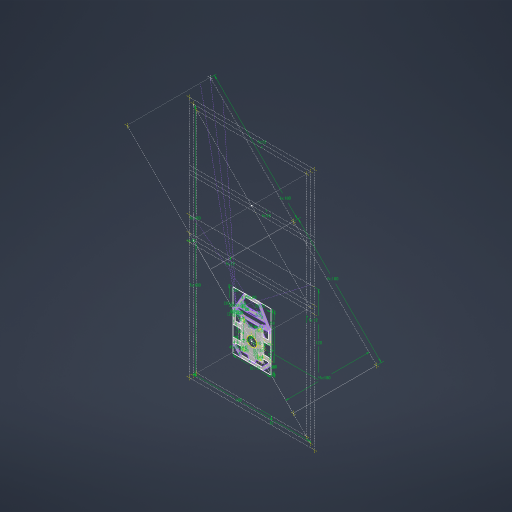
# Autodesk Inventor part: chassis
Saved by Autodesk Inventor 2023.5 (Build 275446000, 446)
## iProperties
Created: 2025-01-19
Part Number: chassis
Material: 一般
Document SubType Name: Modeling
Designer: IshiiLabHonda
Density: 1 g/cm^3
Appearance: 既定
Author: IshiiLabHonda
Autodesk Inventor part; units mm, degrees
ref_plane "YZ Plane" through (0, 0, 0) normal (1, 0, 0) x (0, 1, 0)
ref_plane "XZ Plane" through (0, 0, 0) normal (0, 1, 0) x (-1, 0, 0)
ref_plane "XY Plane" through (0, 0, 0) normal (0, 0, 1) x (1, 0, 0)
sketch "スケッチ1" plane through (0, 0, 0) normal (0, 0, 1) x (1, 0, 0)
  line L0 (-90, 90) -> (90, 90) construction
  line L1 (90, 90) -> (90, -90) construction
  line L2 (90, -90) -> (-90, -90) construction
  line L3 (-90, -90) -> (-90, 90) construction
  line L4 (-90, 90) -> (-90, 270) construction
  line L5 (-90, 270) -> (90, 270) construction
  line L6 (90, 270) -> (90, 90) construction
  line L7 (-90, 90) -> (90, -90) construction
  line L8 (90, 90) -> (-90, -90) construction
  line L9 (0, 0) -> (0, 10) construction
  line L10 (0, 0) -> (10, 0) construction
  line L11 (-90, 270) -> (90, 90) construction
  line L12 (-90, 90) -> (90, 270) construction
  line L13 (-96, 276) -> (96, 276) construction
  line L14 (96, 276) -> (96, -96) construction
  line L15 (96, -96) -> (-96, -96) construction
  line L16 (-96, -96) -> (-96, 276) construction
  line L17 (-84, 264) -> (84, 264) construction
  line L18 (84, 264) -> (84, -84) construction
  line L19 (84, -84) -> (-84, -84) construction
  line L20 (-84, -84) -> (-84, 264) construction
  line L21 (-96, 96) -> (96, 96) construction
  line L22 (-96, 84) -> (96, 84) construction
  line L23 (-63.6396, 63.6396) -> (63.6396, 190.9188) construction
  line L24 (63.6396, 190.9188) -> (190.9188, 63.6396) construction
  line L25 (190.9188, 63.6396) -> (63.6396, -63.6396) construction
  line L26 (63.6396, -63.6396) -> (-63.6396, 63.6396) construction
  line L27 (-190.9188, 190.9188) -> (-63.6396, 318.1981) construction
  line L28 (-63.6396, 318.1981) -> (63.6396, 190.9188) construction
  line L29 (-63.6396, 63.6396) -> (-190.9188, 190.9188) construction
  line L30 (-96, 120) -> (96, 120) construction
  line L31 (-96, 186) -> (96, 186) construction
  line L32 (-96, 174) -> (96, 174) construction
  line L33 (-96, 180) -> (96, 180) construction
  point P0 (-63.6396, 318.1981)
  point P1 (-90, 120)
  point P2 (90, 120)
  point P3 (0, 180)
  dimension "d8" = 10
  dimension "d9" = 10
  dimension "d10" = 12
  dimension "d11" = 12
  dimension "d12" = 12
  dimension "d13" = 12
  dimension "d14" = 180
  dimension "d15" = 180
  dimension "d16" = 180
  dimension "d17" = 12
  dimension "d34" = 180
  dimension "d35" = 180
  dimension "d36" = 180
  dimension "d37" = 120
  dimension "d85" = 12
  constraints: 68 end point, 16 parallel, 16 point on line, 9 perpendicular, 4 midpoint, 3 coincident, 1 horizontal, 7 other
  measures "d8" distance of L9.start L9.end
  measures "d9" distance of L9.start L10.end
  measures "d10" distance between parallel lines of L15 L19
  measures "d11" distance between parallel lines of L16 L20
  measures "d12" distance between parallel lines of L14 L18
  measures "d13" distance between parallel lines of L17 L13
  measures "d14" distance of L1.end L2.end
  measures "d15" distance of L2.end L0.start
  measures "d16" distance between parallel lines of L0 L5
  measures "d17" distance between parallel lines of L22 L21
  measures "d34" distance between parallel lines of L26 L24
  measures "d35" distance of L23.end L24.end
  measures "d36" distance between parallel lines of L23 L27
  measures "d37" distance between parallel lines of L10 L30
  measures "d85" distance between parallel lines of L32 L31
sketch "スケッチ2" plane through (0, 0, 0) normal (0, 0, 1) x (1, 0, 0)
  line L0 (63.6396, 190.9188) -> (190.9188, 63.6396) construction
  line L1 (-63.6396, 318.1981) -> (63.6396, 190.9188) construction
  line L2 (-84, 264) -> (84, 264) construction
  line L3 (-90, 270) -> (90, 270) construction
  line L4 (90, 270) -> (90, 90) construction
  line L5 (-96, 276) -> (96, 276) construction
  line L6 (-90, 90) -> (90, 270) construction
  line L7 (-90, 270) -> (90, 90) construction
  line L8 (-63.6396, 63.6396) -> (63.6396, 190.9188) construction
  line L9 (-96, 120) -> (96, 120) construction
  line L10 (-90, 90) -> (90, 90) construction
  line L11 (-96, 96) -> (96, 96) construction
  line L12 (-96, 84) -> (96, 84) construction
  line L13 (90, -90) -> (-90, -90) construction
  line L14 (0, 0) -> (0, 10) construction
  line L15 (0, 0) -> (10, 0) construction
  line L16 (190.9188, 63.6396) -> (63.6396, -63.6396) construction
  line L17 (63.6396, -63.6396) -> (-63.6396, 63.6396) construction
  line L18 (84, -84) -> (-84, -84) construction
  line L19 (96, -96) -> (-96, -96) construction
  line L20 (-90, 90) -> (-90, 270) construction
  line L21 (-63.6396, 63.6396) -> (-190.9188, 190.9188) construction
  line L22 (-190.9188, 190.9188) -> (-63.6396, 318.1981) construction
  line L23 (96, 276) -> (96, -96) construction
  line L24 (-96, -96) -> (-96, 276) construction
  line L25 (84, 264) -> (84, -84) construction
  line L26 (-84, -84) -> (-84, 264) construction
  line L27 (90, 90) -> (90, -90) construction
  line L28 (-90, 90) -> (90, -90) construction
  line L29 (90, 90) -> (-90, -90) construction
  line L30 (-90, -90) -> (-90, 90) construction
  circle A0 centre (0, 0) radius 16 construction
  circle A1 centre (0, 0) radius 7.5 construction
  line L31 (20, 11.5) -> (28.75, 11.5) construction
  line L32 (28.75, 11.5) -> (28.75, -11.5) construction
  line L33 (28.75, -11.5) -> (20, -11.5) construction
  line L34 (20, -11.5) -> (20, 11.5) construction
  line L35 (20, 11.5) -> (18, 11.5) construction
  line L36 (18, 11.5) -> (18, -11.5) construction
  line L37 (18, -11.5) -> (20, -11.5) construction
  line L38 (18, 1.5) -> (17, 1.5) construction
  line L39 (17, -1.5) -> (18, -1.5) construction
  line L40 (-17, 26) -> (17, 26) construction
  line L41 (17, 26) -> (17, -20) construction
  line L42 (17, -20) -> (-17, -20) construction
  line L43 (-17, -20) -> (-17, 26) construction
  line L44 (-20, 11.5) -> (-28.75, 11.5) construction
  line L45 (-28.75, 11.5) -> (-28.75, -11.5) construction
  line L46 (-28.75, -11.5) -> (-20, -11.5) construction
  line L47 (-20, -11.5) -> (-20, 11.5) construction
  line L48 (-20, 11.5) -> (-18, 11.5) construction
  line L49 (-18, 11.5) -> (-18, -11.5) construction
  line L50 (-18, -11.5) -> (-20, -11.5) construction
  line L51 (-18, 1.5) -> (-17, 1.5) construction
  line L52 (-17, -1.5) -> (-18, -1.5) construction
  line L53 (-14.5, 26) -> (-14.5, -20) construction
  line L54 (14.5, 26) -> (14.5, -20) construction
  line L55 (-10.5, 26) -> (-10.5, 21) construction
  line L56 (-10.5, 21) -> (-14.5, 21) construction
  line L57 (-14.5, 26) -> (-10.5, 21) construction
  line L58 (-10.5, 26) -> (-14.5, 21) construction
  circle A2 centre (-12.5, 23.5) radius 1 construction
  line L59 (10.5, 26) -> (10.5, 21) construction
  line L60 (10.5, 21) -> (14.5, 21) construction
  line L61 (10.5, 26) -> (14.5, 21) construction
  line L62 (10.5, 21) -> (14.5, 26) construction
  circle A3 centre (12.5, 23.5) radius 1 construction
  line L63 (-14.5, -15) -> (-10.5, -15) construction
  line L64 (-10.5, -15) -> (-10.5, -20) construction
  line L65 (10.5, -20) -> (10.5, -15) construction
  line L66 (10.5, -15) -> (14.5, -15) construction
  line L67 (-14.5, -15) -> (-10.5, -20) construction
  line L68 (-10.5, -15) -> (-14.5, -20) construction
  circle A4 centre (-12.5, -17.5) radius 1 construction
  line L69 (10.5, -15) -> (14.5, -20) construction
  line L70 (14.5, -15) -> (10.5, -20) construction
  circle A5 centre (12.5, -17.5) radius 1 construction
  point P0 (90, 120)
  point P1 (-90, 120)
  point P2 (-63.6396, 318.1981)
  point P3 (-12.5, -17.5)
  dimension "d38" = 32
  dimension "d39" = 15
  dimension "d40" = 8.75
  dimension "d41" = 2
  dimension "d42" = 23
  dimension "d44" = 3
  dimension "d45" = 1
  dimension "d48" = 2.5
  dimension "d49" = 20
  dimension "d50" = 26
  dimension "d51" = 2
  dimension "d52" = 5
  dimension "d53" = 4
  dimension "d54" = 2
  dimension "d55" = 4
  dimension "d56" = 5
  dimension "d57" = 2
  dimension "d58" = 4
  dimension "d59" = 5
  dimension "d60" = 2
  dimension "d61" = 5
  dimension "d62" = 4
  dimension "d63" = 57.5
  dimension "d71" = 41
  dimension "d154" = 29
  constraints: 80 end point, 18 point on line, 12 parallel, 10 symmetric about line, 6 centre point, 6 midpoint, 6 perpendicular, 2 coincident, 2 collinear, 5 other
  measures "d38" diameter of A0
  measures "d39" diameter of A1
  measures "d40" distance between parallel lines of L34 L32
  measures "d41" distance between parallel lines of L36 L34
  measures "d42" distance between parallel lines of L33 L31
  measures "d44" distance between parallel lines of L39 L38
  measures "d45" distance between parallel lines of L41 L36
  measures "d48" distance between parallel lines of L43 L53
  measures "d49" distance between parallel lines of L42 L15
  measures "d50" distance between parallel lines of L15 L40
  measures "d51" diameter of A2
  measures "d52" distance of L55.start L55.end
  measures "d53" distance of L55.end L56.end
  measures "d54" diameter of A3
  measures "d55" distance of L59.end L60.end
  measures "d56" distance of L59.start L59.end
  measures "d57" diameter of A4
  measures "d58" distance of L63.start L63.end
  measures "d59" distance of L63.end L64.end
  measures "d60" diameter of A5
  measures "d61" distance of L65.start L65.end
  measures "d62" distance of L65.end L66.end
  measures "d63" distance between parallel lines of L32 L45
  measures "d71" distance of point (-12.5, -17.5) point (-12.5, 23.5)
  measures "d154" distance between parallel lines of L54 L53
sketch "スケッチ3" plane through (0, 0, 0) normal (0, 0, 1) x (1, 0, 0)
  line L0 (63.6396, 190.9188) -> (190.9188, 63.6396) construction
  line L1 (-63.6396, 318.1981) -> (63.6396, 190.9188) construction
  line L2 (-84, 264) -> (84, 264) construction
  line L3 (-90, 270) -> (90, 270) construction
  line L4 (90, 270) -> (90, 90) construction
  line L5 (-96, 276) -> (96, 276) construction
  line L6 (-90, 90) -> (90, 270) construction
  line L7 (-90, 270) -> (90, 90) construction
  line L8 (-63.6396, 63.6396) -> (63.6396, 190.9188) construction
  line L9 (-96, 120) -> (96, 120) construction
  line L10 (-90, 90) -> (90, 90) construction
  line L11 (-96, 96) -> (96, 96) construction
  line L12 (-96, 84) -> (96, 84) construction
  line L13 (90, -90) -> (-90, -90) construction
  line L14 (0, 0) -> (0, 10) construction
  line L15 (0, 0) -> (10, 0) construction
  line L16 (190.9188, 63.6396) -> (63.6396, -63.6396) construction
  line L17 (63.6396, -63.6396) -> (-63.6396, 63.6396) construction
  line L18 (84, -84) -> (-84, -84) construction
  line L19 (96, -96) -> (-96, -96) construction
  line L20 (-90, 90) -> (-90, 270) construction
  line L21 (-63.6396, 63.6396) -> (-190.9188, 190.9188) construction
  line L22 (-190.9188, 190.9188) -> (-63.6396, 318.1981) construction
  line L23 (96, 276) -> (96, -96) construction
  line L24 (-96, -96) -> (-96, 276) construction
  line L25 (84, 264) -> (84, -84) construction
  line L26 (-84, -84) -> (-84, 264) construction
  line L27 (90, 90) -> (90, -90) construction
  line L28 (-90, 90) -> (90, -90) construction
  line L29 (90, 90) -> (-90, -90) construction
  line L30 (-90, -90) -> (-90, 90) construction
  line L31 (-18, 1.5) -> (-17, 1.5) construction
  line L32 (-17, -1.5) -> (-18, -1.5) construction
  line L33 (-20, 11.5) -> (-18, 11.5) construction
  line L34 (-28.75, 11.5) -> (-28.75, -11.5) construction
  line L35 (63.6396, -63.6396) -> (-63.6396, 63.6396) construction
  line L36 (84, -84) -> (-84, -84) construction
  line L37 (-90, -90) -> (-90, 90) construction
  line L38 (96, -96) -> (-96, -96) construction
  line L39 (-90, 90) -> (90, 90) construction
  line L40 (90, -90) -> (-90, -90) construction
  line L41 (90, 90) -> (-90, -90) construction
  line L42 (-90, 90) -> (90, -90) construction
  line L43 (90, 90) -> (90, -90) construction
  line L44 (-28.75, -11.5) -> (-20, -11.5) construction
  line L45 (-20, 11.5) -> (-28.75, 11.5) construction
  line L46 (-18, 11.5) -> (-18, -11.5) construction
  line L47 (-18, -11.5) -> (-20, -11.5) construction
  line L48 (0, 0) -> (0, 10) construction
  line L49 (0, 0) -> (10, 0) construction
  circle A0 centre (0, 0) radius 16 construction
  circle A1 centre (0, 0) radius 7.5 projected
  line L50 (-14.5, 26) -> (-14.5, -20) construction
  line L51 (-17, 26) -> (17, 26) construction
  line L52 (-17, -20) -> (-17, 26) construction
  line L53 (17, -20) -> (-17, -20) construction
  line L54 (-14.5, -15) -> (-10.5, -15) construction
  circle A2 centre (-12.5, -17.5) radius 1 projected
  line L55 (-10.5, -15) -> (-14.5, -20) construction
  line L56 (-14.5, -15) -> (-10.5, -20) construction
  line L57 (-63.6396, 318.1981) -> (63.6396, 190.9188) construction
  line L58 (-84, 264) -> (84, 264) construction
  line L59 (-90, 270) -> (90, 270) construction
  line L60 (90, 270) -> (90, 90) construction
  line L61 (-96, 276) -> (96, 276) construction
  line L62 (-90, 90) -> (90, 270) construction
  line L63 (-90, 270) -> (90, 90) construction
  line L64 (-63.6396, 63.6396) -> (63.6396, 190.9188) construction
  line L65 (-96, 120) -> (96, 120) construction
  line L66 (-96, 96) -> (96, 96) construction
  line L67 (-96, 84) -> (96, 84) construction
  line L68 (84, 264) -> (84, -84) construction
  line L69 (96, 276) -> (96, -96) construction
  line L70 (-96, -96) -> (-96, 276) construction
  line L71 (-84, -84) -> (-84, 264) construction
  line L72 (-63.6396, 63.6396) -> (-190.9188, 190.9188) construction
  line L73 (-90, 90) -> (-90, 270) construction
  line L74 (-190.9188, 190.9188) -> (-63.6396, 318.1981) construction
  line L75 (-20, -11.5) -> (-20, 11.5) construction
  line L76 (10.5, -15) -> (14.5, -15) construction
  line L77 (10.5, -20) -> (10.5, -15) construction
  circle A3 centre (12.5, -17.5) radius 1 projected
  line L78 (10.5, -15) -> (14.5, -20) construction
  line L79 (14.5, -15) -> (10.5, -20) construction
  line L80 (-10.5, -15) -> (-10.5, -20) construction
  line L81 (63.6396, 190.9188) -> (190.9188, 63.6396) construction
  line L82 (190.9188, 63.6396) -> (63.6396, -63.6396) construction
  line L83 (20, 11.5) -> (28.75, 11.5) construction
  line L84 (28.75, 11.5) -> (28.75, -11.5) construction
  line L85 (17, -1.5) -> (18, -1.5) construction
  line L86 (18, -11.5) -> (20, -11.5) construction
  line L87 (28.75, -11.5) -> (20, -11.5) construction
  line L88 (14.5, 26) -> (14.5, -20) construction
  line L89 (17, 26) -> (17, -20) construction
  line L90 (18, 11.5) -> (18, -11.5) construction
  line L91 (20, -11.5) -> (20, 11.5) construction
  line L92 (20, 11.5) -> (18, 11.5) construction
  line L93 (18, 1.5) -> (17, 1.5) construction
  line L94 (-10.5, 26) -> (-10.5, 21) construction
  line L95 (10.5, 21) -> (14.5, 21) construction
  circle A4 centre (12.5, 23.5) radius 1 projected
  line L96 (10.5, 26) -> (14.5, 21) construction
  line L97 (10.5, 21) -> (14.5, 26) construction
  line L98 (10.5, 26) -> (10.5, 21) construction
  line L99 (-10.5, 21) -> (-14.5, 21) construction
  circle A5 centre (-12.5, 23.5) radius 1 projected
  line L100 (-14.5, 26) -> (-10.5, 21) construction
  line L101 (-10.5, 26) -> (-14.5, 21) construction
  line L102 (29.25, 58) -> (29.25, -30)
  line L103 (-29.25, -30) -> (-29.25, 58)
  line L104 (-29.25, 8.5) -> (-17, 8.5)
  line L105 (-17, 8.5) -> (-17, -8.5)
  line L106 (-17, -8.5) -> (-29.25, -8.5)
  line L107 (29.25, 8.5) -> (17, 8.5)
  line L108 (17, 8.5) -> (17, -8.5)
  line L109 (17, -8.5) -> (29.25, -8.5)
  line L110 (10.991, 46.9185) -> (16.1478, 42.9616) construction
  line L111 (11.8865, 37.4081) -> (14.2666, 35.5818) construction
  line L112 (14.2666, 35.5818) -> (18.5279, 41.1353) construction
  line L113 (11.9003, 38.658) -> (10.9773, 45.6686) construction
  line L114 (18.5279, 41.1353) -> (16.1478, 42.9616) construction
  line L115 (11.8865, 37.4081) -> (6.7297, 41.365) construction
  line L116 (11.9003, 38.658) -> (7.9335, 41.7018) construction
  line L117 (7.9335, 41.7018) -> (10.9773, 45.6686) construction
  line L118 (6.7297, 41.365) -> (10.991, 46.9185) construction
  line L119 (10.991, 46.9185) -> (11.8865, 37.4081) construction
  line L120 (14.9441, 42.6248) -> (11.9003, 38.658) construction
  line L121 (7.9335, 41.7018) -> (14.9441, 42.6248) construction
  line L122 (6.7297, 41.365) -> (16.1478, 42.9616) construction
  line L123 (16.1478, 42.9616) -> (11.8865, 37.4081) construction
  line L124 (10.9773, 45.6686) -> (14.9441, 42.6248) construction
  line L125 (-25.2554, 25.0784) -> (-25.9466, 30.0304) construction
  line L126 (-20.1078, 31.6026) -> (-18.8984, 22.9366) construction
  line L127 (-20.9946, 30.7216) -> (-20.3034, 25.7696) construction
  line L128 (-25.2554, 25.0784) -> (-20.9946, 30.7216) construction
  line L129 (-25.9466, 30.0304) -> (-20.3034, 25.7696) construction
  line L130 (-27.0406, 30.635) -> (-20.1078, 31.6026) construction
  line L131 (-18.8984, 22.9366) -> (-25.8312, 21.969) construction
  line L132 (-25.8312, 21.969) -> (-27.0406, 30.635) construction
  line L133 (-63.6396, 318.1981) -> (-23.125, 27.9) construction
  line L134 (11.4388, 42.1633) -> (-90, 120) construction
  line L135 (-23.125, 27.9) -> (-78.8228, 303.0149) construction
  line L136 (-23.125, 27.9) -> (-44.1788, 298.7372) construction
  line L137 (-10.9773, 45.6686) -> (-7.9335, 41.7018) construction
  line L138 (-10.991, 46.9185) -> (-6.7297, 41.365) construction
  line L139 (-16.1478, 42.9616) -> (-10.991, 46.9185) construction
  line L140 (-6.7297, 41.365) -> (-16.1478, 42.9616) construction
  line L141 (-14.9441, 42.6248) -> (-7.9335, 41.7018) construction
  line L142 (-14.9441, 42.6248) -> (-10.9773, 45.6686) construction
  line L143 (-16.1478, 42.9616) -> (-18.5279, 41.1353) construction
  line L144 (-7.9335, 41.7018) -> (-11.9003, 38.658) construction
  line L145 (-10.9773, 45.6686) -> (-11.9003, 38.658) construction
  line L146 (-11.9003, 38.658) -> (-14.9441, 42.6248) construction
  line L147 (-10.991, 46.9185) -> (-11.8865, 37.4081) construction
  line L148 (-6.7297, 41.365) -> (-11.8865, 37.4081) construction
  line L149 (-11.8865, 37.4081) -> (-16.1478, 42.9616) construction
  line L150 (-18.5279, 41.1353) -> (-14.2666, 35.5818) construction
  line L151 (-14.2666, 35.5818) -> (-11.8865, 37.4081) construction
  line L152 (-11.4388, 42.1633) -> (90, 120) construction
  circle A6 centre (-8.395, 38.1965) radius 0.625 construction
  circle A7 centre (-8.395, 38.1965) radius 0.8
  circle A8 centre (-8.395, 38.1965) radius 1.5 construction
  circle A9 centre (-15.2072, 39.2717) radius 0.625 construction
  circle A10 centre (-15.2072, 39.2717) radius 0.8
  circle A11 centre (-15.2072, 39.2717) radius 1.5 construction
  line L153 (-20.3034, 25.7696) -> (-25.2554, 25.0784) construction
  line L154 (-26.1422, 24.1974) -> (-19.2094, 25.165) construction
  line L155 (-25.601, 27.5544) -> (-20.649, 28.2456) construction
  line L156 (-22.3648, 22.4528) -> (-22.7794, 25.424) construction
  circle A12 centre (-18.173, 28.5911) radius 1.5 construction
  circle A13 centre (-18.173, 28.5911) radius 0.8
  circle A14 centre (-18.173, 28.5911) radius 0.625 construction
  circle A15 centre (-27.1405, 25.3286) radius 0.8
  circle A16 centre (-27.1405, 25.3286) radius 0.625 construction
  line L157 (-25.9466, 30.0304) -> (-20.9946, 30.7216) construction
  circle A17 centre (8.395, 38.1965) radius 0.625 construction
  circle A18 centre (8.395, 38.1965) radius 0.8
  circle A19 centre (8.395, 38.1965) radius 1.5 construction
  circle A20 centre (15.2072, 39.2717) radius 1.5 construction
  circle A21 centre (15.2072, 39.2717) radius 0.8
  circle A22 centre (15.2072, 39.2717) radius 0.625 construction
  circle A23 centre (18.173, 28.5911) radius 0.625 construction
  circle A24 centre (18.173, 28.5911) radius 0.8
  circle A25 centre (18.173, 28.5911) radius 1.5 construction
  circle A26 centre (27.1405, 25.3286) radius 0.625 construction
  circle A27 centre (27.1405, 25.3286) radius 0.8
  circle A28 centre (27.1405, 25.3286) radius 1.5 construction
  line L158 (-29.25, -30) -> (29.25, -30)
  line L159 (-29.25, 58) -> (29.25, 58)
  line L160 (-11.4388, 42.1633) -> (-8.395, 38.1965) construction
  line L161 (-29.25, 28.2016) -> (-12.0459, 58)
  line L162 (-29.25, -17.6878) -> (-16.9378, -30)
  line L163 (29.25, 28.2016) -> (12.0459, 58)
  line L164 (29.25, -17.6878) -> (16.9378, -30)
  line L165 (-9.7365, 54) -> (9.7365, 54)
  line L166 (9.7365, 54) -> (25.25, 27.1298)
  line L167 (25.25, 27.1298) -> (25.25, 14.5)
  line L168 (25.25, 14.5) -> (17, 14.5)
  line L169 (3.695, 18.0905) -> (-3.695, 18.0905)
  line L170 (-17, 14.5) -> (-25.25, 14.5)
  line L171 (-25.25, 14.5) -> (-25.25, 27.1298)
  line L172 (-25.25, 27.1298) -> (-9.7365, 54)
  line L173 (20.1078, 31.6026) -> (18.8984, 22.9366) construction
  line L174 (20.9946, 30.7216) -> (20.3034, 25.7696) construction
  line L175 (25.9466, 30.0304) -> (20.3034, 25.7696) construction
  line L176 (25.2554, 25.0784) -> (20.9946, 30.7216) construction
  line L177 (27.0406, 30.635) -> (20.1078, 31.6026) construction
  line L178 (25.2554, 25.0784) -> (25.9466, 30.0304) construction
  line L179 (18.8984, 22.9366) -> (25.8312, 21.969) construction
  line L180 (25.8312, 21.969) -> (27.0406, 30.635) construction
  line L181 (20.3034, 25.7696) -> (25.2554, 25.0784) construction
  line L182 (26.1422, 24.1974) -> (19.2094, 25.165) construction
  line L183 (25.9466, 30.0304) -> (20.9946, 30.7216) construction
  line L184 (-9.7365, 22.9366) -> (-9.7365, 26)
  line L185 (9.7365, 22.9366) -> (9.7365, 26)
  line L186 (9.7365, 26) -> (17, 26)
  line L187 (17, 26) -> (17, 14.5)
  line L188 (-9.7365, 26) -> (-17, 26)
  line L189 (-17, 26) -> (-17, 14.5)
  line L190 (-9.7365, 22.9366) -> (-3.695, 18.0905)
  line L191 (9.7365, 22.9366) -> (3.695, 18.0905)
  line L192 (-17, -14.5) -> (-25.25, -14.5)
  line L193 (-25.25, -14.5) -> (-25.25, -16.0309)
  line L194 (-25.25, -16.0309) -> (-15.2809, -26)
  line L195 (-15.2809, -26) -> (15.2809, -26)
  line L196 (15.2809, -26) -> (25.25, -16.0309)
  line L197 (25.25, -16.0309) -> (25.25, -14.5)
  line L198 (25.25, -14.5) -> (17, -14.5)
  line L199 (17, -14.5) -> (17, -20.8804)
  line L200 (17, -20.8804) -> (6.6466, -20.8804)
  line L201 (6.6466, -20.8804) -> (4.5158, -27.0126)
  line L202 (4.5158, -27.0126) -> (-4.5158, -27.0126)
  line L203 (-4.5158, -27.0126) -> (-6.6466, -20.8804)
  line L204 (-6.6466, -20.8804) -> (-17, -20.8804)
  line L205 (-17, -20.8804) -> (-17, -14.5)
  line L206 (-16.1661, 42.8636) -> (16.1661, 42.8636)
  line L207 (-20.6579, 35.0836) -> (20.6579, 35.0836)
  line L208 (-22.045, 32.6811) -> (-12.2942, 28.5594)
  line L209 (-12.2942, 28.5594) -> (12.2942, 28.5594)
  line L210 (12.2942, 28.5594) -> (22.045, 32.6811)
  line L211 (-25.25, 25.1515) -> (25.25, 25.1515)
  circle A29 centre (-27.1405, 25.3286) radius 1.5 construction
  line L212 (-7.5571, 35.0836) -> (-5.0762, 37.1727)
  line L213 (-5.0762, 37.1727) -> (5.0762, 37.1727)
  line L214 (5.0762, 37.1727) -> (7.5571, 35.0836)
  line L215 (-6.2476, 42.8636) -> (0, 41.1322)
  line L216 (0, 41.1322) -> (6.2476, 42.8636)
  line L217 (-17, 18.9574) -> (-20.6579, 14.5)
  line L218 (17, 18.9574) -> (20.6579, 14.5)
  point P0 (29.25, -8.5)
  point P1 (29.25, 8.5)
  point P2 (29.25, -17.6878)
  point P3 (29.25, 28.2016)
  point P4 (16.5079, 42.2717)
  point P5 (9.7365, 25.1515)
  point P6 (-9.7365, 25.1515)
  point P7 (17, 25.1515)
  point P8 (-17, 25.1515)
  point P9 (-4.3925, 58)
  point P10 (4.5158, 58)
  point P11 (4.8676, -26)
  point P12 (-4.8676, -26)
  dimension "d78" = 17
  dimension "d80" = 0.5
  dimension "d81" = 58.5
  dimension "d82" = 57.5
  dimension "d84" = 0
  dimension "d119" = 5
  dimension "d123" = 5
  dimension "d124" = 5
  dimension "d125" = 6.5
  dimension "d126" = 7
  dimension "d127" = 3
  dimension "d128" = 7
  dimension "d130" = 5
  dimension "d131" = 5
  dimension "d132" = 6.5
  dimension "d133" = 7
  dimension "d134" = 3
  dimension "d135" = 105
  dimension "d141" = 1.25
  dimension "d142" = 1.6
  dimension "d143" = 3
  dimension "d144" = 1.25
  dimension "d145" = 1.6
  dimension "d146" = 3
  dimension "d156" = 3
  dimension "d157" = 6.5
  dimension "d158" = 7
  dimension "d161" = 1.25
  dimension "d162" = 1.6
  dimension "d163" = 3
  dimension "d164" = 1.25
  dimension "d165" = 1.6
  dimension "d173" = 5
  dimension "d187" = 88
  dimension "d192" = 2.2094
  dimension "d193" = 58
  dimension "d194" = 30
  dimension "d195" = 30.1
  dimension "d198" = 45
  dimension "d199" = 30
  dimension "d203" = 4
  dimension "d204" = 4
  dimension "d205" = 0
  dimension "d206" = 4
  dimension "d207" = 4
  dimension "d208" = 4
  dimension "d209" = 4
  dimension "d210" = 6
  dimension "d211" = 6
  dimension "d240" = 3
  constraints: 234 end point, 48 horizontal alignment, 37 parallel, 35 point on line, 27 perpendicular, 24 centre point, 17 coincident, 14 midpoint, 11 equal radius, 6 horizontal, 3 tangent, 1 equal length, 18 other
  measures "d78" distance between parallel lines of L106 L104
  measures "d80" distance between parallel lines of L103 L34
  measures "d81" distance between parallel lines of L102 L103
  measures "d82" distance between parallel lines of L84 L34
  measures "d84" distance between parallel lines of L105 L52
  measures "d119" distance between parallel lines of L125 L127
  measures "d123" distance between parallel lines of L120 L117
  measures "d124" distance of L124.end L113.start
  measures "d125" distance between parallel lines of L123 L118
  measures "d126" distance between parallel lines of L110 L115
  measures "d127" distance between parallel lines of L112 L123
  measures "d128" angle of L135 L136
  measures "d130" distance between parallel lines of L146 L137
  measures "d131" distance of L144.end L141.start
  measures "d132" distance between parallel lines of L149 L138
  measures "d133" distance between parallel lines of L148 L139
  measures "d134" distance between parallel lines of L150 L149
  measures "d135" angle of L134 L152
  measures "d141" diameter of A6
  measures "d142" diameter of A7
  measures "d143" diameter of A8
  measures "d144" diameter of A9
  measures "d145" diameter of A10
  measures "d146" diameter of A11
  measures "d156" distance between parallel lines of L131 L153
  measures "d157" distance between parallel lines of L154 L130
  measures "d158" distance between parallel lines of L126 L132
  measures "d161" diameter of A14
  measures "d162" diameter of A13
  measures "d163" diameter of A12
  measures "d164" diameter of A16
  measures "d165" diameter of A15
  measures "d173" distance of L128.start L129.start
  measures "d187" distance between parallel lines of L158 L159
  measures "d192" distance from line of L103 L130.start
  measures "d193" distance of the line from the sketch origin of L159
  measures "d194" distance of the line from the sketch origin of L158
  measures "d195" distance from line of point (-23.125, 27.9) L159
  measures "d198" angle of L103 L162
  measures "d199" angle of L103 L161
  measures "d203" distance between parallel lines of L165 L159
  measures "d204" distance between parallel lines of L161 L172
  measures "d205" distance between parallel lines of L189 L52
  measures "d206" distance between parallel lines of L103 L171
  measures "d207" distance between parallel lines of L158 L195
  measures "d208" distance between parallel lines of L162 L194
  measures "d209" distance between parallel lines of L103 L193
  measures "d210" distance between parallel lines of L192 L106
  measures "d211" distance between parallel lines of L104 L170
  measures "d240" diameter of A29
extrude "押し出し1" add sketch "スケッチ3" against normal blind 1 contours A1 | A2 | A3 | A4 | A5 | L102 L163 L159 | L102 L107 L108 L109 L164 L158 L162 L103 L106 L105 L104 L161 L159 L163 | L102 L109 L108 L107 | L161 L103 L159 | L102 L158 L164 | L104 L105 L106 L103 | L158 L103 L162 | A7 | A10 | A13 | A15 | A18 | A21 | A24 | A27 | L165 L166 L206 L172 | L206 L215 L216 L166 L207 L214 L213 L212 L172 | L207 L166 L210 L209 L208 L172 | L206 L216 L215 | L208 L209 L210 L166 L167 L211 L187 L186 L185 L184 L188 L189 L171 L172 | L212 L213 L214 L207 | L211 L189 L217 L170 L171 | L167 L168 L218 L187 L211 | L189 L188 L184 L211 | L211 L185 L186 L187 | L217 L189 L170 | L211 L185 L191 L169 L190 L184 | L168 L187 L218 | L205 L204 L203 L195 L194 L193 L192 | L201 L200 L199 L198 L197 L196 L195 | L195 L201 L202 L203
extrude "押し出し2" cut sketch "スケッチ3" against normal blind 1 contours A2 | A3 | A4 | A5
extrude "押し出し3" cut sketch "スケッチ3" against normal blind 1 contours A1
extrude "押し出し4" cut sketch "スケッチ3" against normal up to surface (1 mm away) contours L102 L109 L108 L107 | L104 L105 L106 L103
extrude "押し出し7" cut sketch "スケッチ3" against normal up to surface (1 mm away) contours A7 | A10 | A18 | A21 | A24 | A27
extrude "押し出し8" cut sketch "スケッチ3" against normal blind 10 contours A13 | A15
extrude "押し出し24" cut sketch "スケッチ3" against normal blind 1 contours L102 L163 L159 | L161 L103 L159 | L102 L158 L164 | L158 L103 L162 | L165 L166 L206 L172 | L207 L166 L210 L209 L208 L172 | L206 L216 L215 | L212 L213 L214 L207 | L211 L189 L217 L170 L171 | L167 L168 L218 L187 L211 | L217 L189 L170 | L211 L185 L191 L169 L190 L184 | L168 L187 L218 | L205 L204 L203 L195 L194 L193 L192 | L201 L200 L199 L198 L197 L196 L195
extrude "押し出し27" add sketch "スケッチ3" against normal blind 1 contours L217 L189 L170 | L168 L187 L218
chamfer "面取り3" distance 2 angle 45 4 edges at (-29.25, 8.5, -0.5) (-29.25, -8.5, -0.5) (29.25, -8.5, -0.5) (29.25, 8.5, -0.5)
chamfer "面取り4" distance 5 angle 45 2 edges at (-16.1661, 42.8636, -0.5) (16.1661, 42.8636, -0.5)
chamfer "面取り5" distance 2 angle 45 2 edges at (17, -14.5, -0.5) (-17, -14.5, -0.5)
chamfer "面取り6" distance 2 angle 45 2 edges at (17, -20.8804, -0.5) (-17, -20.8804, -0.5)
chamfer "面取り7" distance 2 angle 45 2 edges at (4.8676, -26, -0.5) (-4.8676, -26, -0.5)
equation "\"d9\" = d8"
equation "\"d11\" = d10"
equation "\"d12\" = d10"
equation "\"d13\" = d10"
equation "\"d15\" = d14"
equation "\"d16\" = d14"
equation "\"d17\" = d10"
